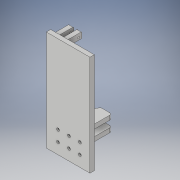
# Autodesk Inventor part: Verbinder_Tisch_Dewar
Saved by Autodesk Inventor 2019 (Build 230136000, 136)
## iProperties
Created: 2018-09-27
Part Number: Verbinder_Tisch_Dewar
Material: Generic
Document SubType Name: Modeling
Designer: Q
Density: 1 g/cm^3
Appearance: Default
d0: 10,000 mm
d1: 0,00 deg
d2: 6,600 mm
d4: 11,000 mm
d5: 6,800 mm
d10: 5,000 mm
d11: 20,000 mm
d13: 60,00 deg
d14: 5,000 mm
d15: 10,000 mm
d16: 0,00 deg
d18: 4,200 mm
d19: 10,000 mm
d20: 50,000 mm
d21: 0,00 deg
d22: 5,000 mm
d23: 15,750 mm
d24: 0,00 deg
d25: 50,000 mm
d26: 35,000 mm
d27: 5,000 mm
d28: 7,000 mm
d29: 0,00 deg
d30: 13,500 mm
d35: 32,300 mm
d36: 118,00 deg
d48: 13,500 mm
d49: 2,000 mm
d50: 10,000 mm
d51: 0,00 deg
d52: 100,000 mm
d53: 55,000 mm
d54: 15,000 mm
d55: 0,00 deg
d17: 4,200 mm
Author: Q
Autodesk Inventor part; units mm, degrees
ref_plane "Work Plane1" through (-166.5525, 2.666, -98.7961) normal (0, 0, -1) x (-1, 0, 0)
sketch "Sketch1" plane through (-166.5525, 2.666, -98.7961) normal (0, 0, -1) x (-1, 0, 0)
  line L0 (-233.1482, 205) -> (-133.1482, 205)
  line L1 (-133.1482, 205) -> (-133.1482, -25)
  line L2 (-133.1482, -25) -> (-233.1482, -25)
  line L3 (-233.1482, -25) -> (-233.1482, 205)
  circle A0 centre (0, 0) radius 140 projected
  circle A1 centre (-210, 25) radius 2.4585 projected
  circle A2 centre (-185, 25) radius 2.4585 projected
  circle A3 centre (-160, 25) radius 2.4585 projected
  circle A4 centre (-185, 0) radius 2.4585 projected
  circle A5 centre (-210, 0) radius 2.4585 projected
  circle A6 centre (-160, 0) radius 2.4585 projected
  circle A7 centre (0.3518, 0) radius 128.5 projected
  line L4 (-128.1482, 39.0483) -> (-128.1482, -22.9652) construction
  dimension "d10" = 5
  dimension "d56" = 230
  dimension "d57" = 100
  dimension "d63" = 25
  constraints: 10 end point, 2 parallel, 1 horizontal, 1 perpendicular, 1 tangent
  measures "d10" distance between parallel lines of L1 L4
  measures "d56" distance between parallel lines of L2 L0
  measures "d57" distance of L0.start L0.end
  measures "d63" distance from line of L2 A6.centre
extrude "Extrusion1" add sketch "Sketch1" along normal blind 10 contours L0 L1 A0 L2 L3 | L1 L2 A0 | A1 | A2 | A3 | A4 | A5 | A6 picked at (-134.3536, 16.0623)
hole "Hole1" at (43.4475, 27.666, -108.7961) at (18.4475, 27.666, -108.7961) at (-6.5525, 27.666, -108.7961) at (43.4475, 2.666, -108.7961) at (18.4475, 2.666, -108.7961) at (-6.5525, 2.666, -108.7961) direction (0, 0, 1) diameter 6.6 end through all counterbore diameter 11 counterbore depth 6.8 clearance for "Socket Head Cap Screw ISO 4762" size "M6" standard "ISO"
ref_plane "Work Plane2" through (-38.4044, -9.834, -118.7961) normal (0, -1, 0) x (1, 0, 0)
sketch "Sketch3" plane through (-38.4044, -9.834, -118.7961) normal (0, -1, 0) x (1, 0, 0)
  line L0 (5, 10) -> (55, 10)
  line L1 (55, 10) -> (55, -75)
  line L2 (50, -80) -> (32.7284, -80)
  line L3 (5, -35.6333) -> (5, 10)
  line L4 (105, 10) -> (5, 10) projected
  line L5 (5, 20) -> (5, 10) projected
  circle A0 centre (22.225, -22.225) radius 12.7 projected
  circle A1 centre (22.225, -22.225) radius 10
  line L6 (5.6699, -38.1333) -> (28.3983, -77.5)
  line L7 (5, -36.973) -> (50.4568, -36.973) construction
  arc A2 (28.3983, -77.5) -> (32.7284, -80) centre (32.7284, -75) ccw
  arc A3 (50, -80) -> (55, -75) centre (50, -75) ccw
  arc A4 (5, -35.6333) -> (5.6699, -38.1333) centre (10, -35.6333) ccw
  point P0 (38.4044, 118.7961)
  dimension "d11" = 20
  dimension "d13" = 60
  dimension "d14" = 5
  dimension "d58" = 90
  dimension "d60" = 50
  constraints: 12 end point, 6 point on circle, 6 tangent, 4 centre point, 2 collinear, 2 equal radius, 2 horizontal, 2 parallel, 2 point on line, 1 coincident, 1 equal length, 1 perpendicular
  measures "d11" diameter of A1
  measures "d13" angle of L6 L7
  measures "d14" radius of A2
  measures "d58" distance between parallel lines of L4 L2
  measures "d60" distance of L0.start L0.end
extrude "Extrusion2" add sketch "Sketch3" along normal mid plane 10 contours L0 L1 A3 L2 A2 L6 A4 L3 | A0
ref_plane "Work Plane3" through (-25.7044, 2.666, -220.3961) normal (0, -1, 0) x (1, 0, 0)
mirror "Mirror1" about plane through (-25.7044, 2.666, -220.3961) normal (0, -1, 0) of "Extrusion2"
sketch "Sketch4" plane through (-166.5525, 2.666, -108.7961) normal (0, 0, -1) x (-1, 0, 0)
  line L0 (-133.1482, 205) -> (-133.1482, -25) projected
  line L1 (-133.1482, 32.5) -> (-183.1482, 32.5)
  line L2 (-183.1482, 32.5) -> (-183.1482, 42.5)
  line L3 (-183.1482, 42.5) -> (-133.1482, 42.5)
  line L4 (-133.1482, 42.5) -> (-133.1482, 32.5)
  line L5 (-183.1482, 17.5) -> (-183.1482, 7.5) projected
  circle A0 centre (-185, 25) radius 3.3 projected
  line L6 (-160.8766, 17.5) -> (-178.1482, 17.5) projected
  point P0 (-166.5525, -2.666)
  dimension "d17" = 4.2
  dimension "d18" = 4.2
  dimension "d19" = 10
  constraints: 8 end point, 2 parallel, 1 collinear, 1 horizontal, 1 perpendicular, 1 point on line
  measures "d17" distance edge to line of A0 L6
  measures "d18" distance edge to line of A0 L1
  measures "d19" distance between parallel lines of L3 L1
extrude "Extrusion3" add sketch "Sketch4" along normal blind 50 contours L0 L1 L2 L3
fillet "Fillet1" radius 5 2 edges at (-33.4044, 40.166, -158.7961) (16.5956, 40.166, -158.7961)
sketch "Sketch5" plane through (-33.4044, 45.166, -108.7961) normal (0, 1, 0) x (1, 0, 0)
  circle A0 centre (17.225, 32.225) radius 10 projected
  point P0 (33.4044, -108.7961)
extrude "Extrusion4" cut sketch "Sketch5" against normal blind 15.75
ref_plane "Work Plane6" through (-16.1794, 92.1501, -148.7711) normal (0, -1, 0) x (0, 0, 1)
sketch "Sketch7" plane through (-16.1794, 92.1501, -148.7711) normal (0, -1, 0) x (0, 0, 1)
  line L0 (39.975, 17.225) -> (39.975, -82.775) projected
  line L1 (39.975, 17.225) -> (-5.025, 17.225)
  line L2 (-10.025, 12.225) -> (-10.025, -12.775)
  line L3 (-5.025, -17.775) -> (39.975, -17.775)
  line L4 (39.975, -17.775) -> (39.975, 17.225)
  arc A0 (-5.025, 17.225) -> (-10.025, 12.225) centre (-5.025, 12.225) ccw
  arc A1 (-10.025, -12.775) -> (-5.025, -17.775) centre (-5.025, -12.775) ccw
  point P0 (148.7711, -16.1794)
  point P1 (-10.025, -17.775)
  point P2 (-10.025, 17.225)
  point P3 (7.75, 0)
  dimension "d25" = 50
  dimension "d26" = 35
  dimension "d27" = 5
  constraints: 8 end point, 4 point on circle, 4 point on line, 4 tangent, 2 centre point, 2 parallel, 1 equal radius, 1 horizontal, 1 perpendicular
  measures "d25" distance of L3.end point (-10.025, -17.775)
  measures "d26" distance of point (-10.025, -17.775) point (-10.025, 17.225)
  measures "d27" radius of A0
extrude "Extrusion5" [suppressed]
sketch "Sketch8" plane through (-16.1794, 85.1501, -148.7711) normal (0, -1, 0) x (1, 0, 0)
  point P0 (16.1794, 148.7711)
  point P1 (0, 7.75)
hole "Hole2" [suppressed]
ref_plane "Work Plane8" through (-11.7294, 189.1501, -141.0211) normal (1, 0, 0) x (0, -1, 0)
sketch "Sketch12" plane through (-11.7294, 189.1501, -141.0211) normal (1, 0, 0) x (0, -1, 0)
  circle A0 centre (-2, 0) radius 2 projected
  line L0 (0, 4.5164) -> (0, 7) projected
  line L1 (-9.233, 4.5164) -> (0, 4.5164) projected
  spline S0 degree 2 poles (-10, 3.4325) (-9.6688, 3.9374) (-9.233, 4.5164) knots 0 0 0 0.1328 0.1328 0.1328 weights 1 1.004688 1 projected
  line L2 (-10, -3.4325) -> (-10, 3.4325) projected
  spline S1 degree 2 poles (-9.233, -4.5164) (-9.6688, -3.9374) (-10, -3.4325) knots 0 0 0 0.1328 0.1328 0.1328 weights 1 1.004688 1 projected
  line L3 (0, -4.5164) -> (-9.233, -4.5164) projected
  line L4 (0, -7) -> (0, -4.5164) projected
  line L5 (0, -7) -> (4.2876, -7) projected
  spline S2 degree 2 poles (4, -6.6678) (4.1403, -6.8309) (4.2876, -7) knots 0 0 0 0.044596 0.044596 0.044596 weights 1 1.000378 1.000314 projected
  line L6 (4, 6.6678) -> (4, -6.6678) projected
  spline S3 degree 2 poles (4.2876, 7) (4.1403, 6.8309) (4, 6.6678) knots 0.03161 0.03161 0.03161 0.076206 0.076206 0.076206 weights 1.000314 1.000378 1 projected
  line L7 (-18.5159, -32.225) -> (211.4841, -32.225) projected
  line L8 (1.2341, 7.775) -> (-8.2659, 7.775)
  line L9 (-10.2659, 5.775) -> (-10.2659, -32.225)
  line L10 (-10.2659, -32.225) -> (3.2341, -32.225)
  line L11 (3.2341, -32.225) -> (3.2341, 5.775)
  arc A1 (-8.2659, 7.775) -> (-10.2659, 5.775) centre (-8.2659, 5.775) ccw
  arc A2 (3.2341, 5.775) -> (1.2341, 7.775) centre (1.2341, 5.775) ccw
  line L12 (-18.5159, -42.225) -> (-18.5159, -32.225) projected
  point P0 (189.1501, -141.0211)
  point P1 (3.2341, 7.775)
  point P2 (-3.5159, 7.775)
  dimension "d48" = 13.5
  dimension "d49" = 2
  dimension "d62" = 40
  dimension "d79" = 15
  constraints: 8 end point, 4 point on circle, 4 tangent, 3 point on line, 2 centre point, 2 parallel, 1 equal radius, 1 horizontal, 1 midpoint, 1 perpendicular
  measures "d48" distance between parallel lines of L11 L9
  measures "d49" radius of A1
  measures "d62" distance between parallel lines of L10 L8
  measures "d79" distance from line of L12 point (-3.516, 7.775)
extrude "Extrusion7" add sketch "Sketch12" along normal blind 10
ref_plane "Work Plane10" through (-16.1794, 180.6501, -141.0211) normal (-1, 0, 0) x (0, 1, 0)
ref_plane "Work Plane9" through (-20.6294, 180.6501, -141.0211) normal (-1, 0, 0) x (0, 1, 0)
mirror "Mirror2" about plane through (-16.1794, 180.6501, -141.0211) normal (-1, 0, 0) of "Extrusion7"
sketch "Sketch13" plane through (-166.5525, 2.666, -108.7961) normal (0, 0, -1) x (-1, 0, 0)
  line L0 (-233.1482, 205) -> (-188.1482, 205)
  line L1 (-188.1482, 205) -> (-188.1482, 75)
  line L2 (-188.1482, 75) -> (-233.1482, 75)
  line L3 (-233.1482, 75) -> (-233.1482, 205)
  line L4 (-233.1482, -25) -> (-133.1482, -25) projected
  line L5 (-133.1482, 42.5) -> (-133.1482, 205) projected
  point P0 (-166.5525, -2.666)
  point P1 (-133.1482, 89.4841)
  dimension "d52" = 100
  dimension "d53" = 55
  constraints: 8 end point, 2 parallel, 1 horizontal, 1 perpendicular
  measures "d52" distance between parallel lines of L4 L2
  measures "d53" distance between parallel lines of L5 L1
extrude "Extrusion8" [suppressed]
ref_plane "Work Plane11" through (-33.4044, 2.666, -108.7961) normal (0, -1, 0) x (1, 0, 0)
sketch "Sketch15" plane through (-166.5525, 2.666, -108.7961) normal (0, 0, -1) x (-1, 0, 0)
  line L0 (-133.1482, 205) -> (-133.1482, -25) construction
  line L1 (-133.1482, 95) -> (-183.1482, 95) construction
  line L2 (-133.1482, 95) -> (-83.1482, 95) construction
  line L3 (-133.1482, 205) -> (-233.1482, 205) construction
  line L4 (-183.1482, 91.5) -> (-133.1482, 91.5)
  line L5 (-133.1482, 91.5) -> (-133.1482, 98.5)
  line L6 (-133.1482, 98.5) -> (-183.1482, 98.5)
  line L7 (-183.1482, 98.5) -> (-183.1482, 91.5)
  line L8 (-183.1482, 91.5) -> (-133.1482, 98.5) construction
  line L9 (-133.1482, 91.5) -> (-183.1482, 98.5) construction
  point P0 (-166.5525, -2.666)
  point P1 (-158.1482, 95)
  dimension "d64" = 50
  dimension "d65" = 180
  dimension "d66" = 110
  dimension "d67" = 7
  constraints: 16 end point, 3 midpoint, 2 horizontal, 2 parallel, 2 perpendicular, 2 point on line, 1 collinear
  measures "d64" distance of L1.start L1.end
  measures "d65" angle of L1 L2
  measures "d66" distance between parallel lines of L3 L1
  measures "d67" distance of L5.end L4.end
extrude "Extrusion9" add sketch "Sketch15" along normal blind 50
fillet "Fillet2" radius 5 2 edges at (-33.4044, 97.666, -158.7961) (16.5956, 97.666, -158.7961)
sketch "Sketch16" plane through (-33.4044, 101.166, -108.7961) normal (0, 1, 0) x (1, 0, 0)
  point P0 (33.4044, -108.7961)
  point P1 (17.225, 32.225)
hole "Hole3" at (-16.1794, 101.166, -141.0211) direction (0, -1, 0) diameter 12.2 depth 17.1 tip angle 118
equation "\"d18\" = d17"
body "Solid1"
